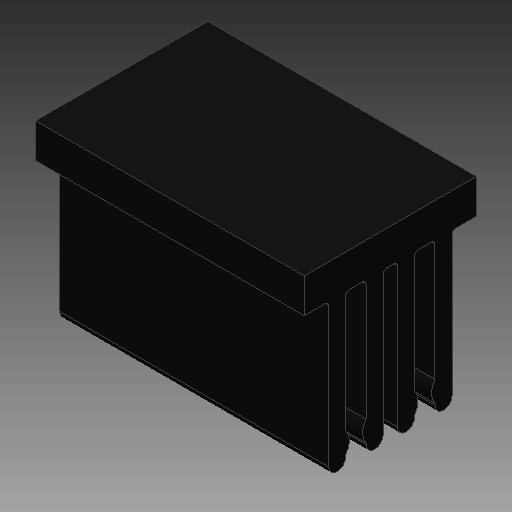
# Autodesk Inventor part: PPP-06-01-20--DV
Saved by Autodesk Inventor 2019.1 (Build 231200000, 200)
## iProperties
Category: PARTsolutions
Company: SAMTEC
Created: 2015-08-01
Part Number: PPP-06-01-20--DV
Catalog Web Link: www.cadenas.de
Description: TSM Series Pick & Place Pad-TSM Series - (2,54 mm) .100" Surface Mount Terminal .025" Square Post Header
Vendor: SAMTEC
Document SubType Name: Modeling
Designer: PARTuser1
Manufacturer: SAMTEC
Mass: 0.221539 g
Surface Area: 6.25221 cm^2
Volume: 0.221539 cm^3
Density: 1 g/cm^3
Material: Allgemein
Appearance: PSOLRGB-0-0-0
PSOL_IDENT_0: {$CADENAS_DATA\23d-libs\samtec\modelling\tsm\parts\tsm_ppp.prj},205 {VTYP=3D},{NB=PPP-06-01-20--DV},
PSOL_IDENT_1: {LINA=PPP-06-01-20--DV},{NN=TSM Series Pick & Place Pad},{DATE=15.05.2015 12:28:13},{GEOMDATE=25.09.
PSOL_IDENT_2: 2014 07:23:00},{VERSION=},{LINEID=10},{LINESUBID=-1},{WBVAR=LS,POS,ROW}  {NB=PPP-06-01-20--DV},{LINA=
PSOL_IDENT_3: PPP-06-01-20--DV},{KT=DUMMY},{PN=PPP-06-01-20--DV},{LS=-01},{POS=20},{ROW=-DV},{BSH=0.230},{CSH=0.18
PSOL_IDENT_4: 0},{ESH=0.1000},{ASH=0.9000},{POSOE=2},{BSV=0.230},{CSV=0.2800}
NN: TSM Series Pick & Place Pad
NT: TSM Series - (2,54 mm) .100" Surface Mount Terminal .025" Square Post Header
NB: PPP-06-01-20--DV
NBSYN: $PN.
LINA: PPP-06-01-20--DV
LS: -01
POS: 20
ROW: -DV - Double Vertical
SUPPLIER: SAMTEC
ARTICLENO: PPP-06-01-20--DV
BOMINFO: PPP-06-01-20--DV
CREATOR: CADENAS GmbH
Title: PPP-06-01-20--DV
Author: Cadenas PARTsolutions
Comments: TSM Series - (2,54 mm) .100" Surface Mount Terminal .025" Square Post Header
Autodesk Inventor part; units mm, degrees
sketch "Sketch_6" plane through (0, 0, 0) normal (1, 0, 0) x (0, 1, 0)
  line L0 (0, 3.175) -> (-1.27, 3.175)
  line L1 (-1.27, 3.175) -> (-1.27, 2.407)
  arc A0 (-1.397, 2.28) -> (-1.27, 2.407) centre (-1.397, 2.407) ccw
  line L2 (-1.397, 2.28) -> (-6.54, 2.28)
  arc A1 (-6.54, 2.28) -> (-6.54, 1.645) centre (-6.54, 1.9625) ccw
  line L3 (-6.54, 1.645) -> (-6.477, 1.645)
  arc A2 (-6.477, 1.645) -> (-5.715, 1.645) centre (-6.096, 2.153) ccw
  line L4 (-5.715, 1.645) -> (-1.397, 1.645)
  arc A3 (-1.27, 1.518) -> (-1.397, 1.645) centre (-1.397, 1.518) ccw
  line L5 (-1.27, 1.518) -> (-1.27, 1.022)
  arc A4 (-1.397, 0.895) -> (-1.27, 1.022) centre (-1.397, 1.022) ccw
  line L6 (-1.397, 0.895) -> (-5.715, 0.895)
  arc A5 (-5.715, 0.895) -> (-6.477, 0.895) centre (-6.096, 0.387) ccw
  line L7 (-6.477, 0.895) -> (-6.5222, 0.895)
  arc A6 (-6.5222, 0.895) -> (-6.5222, 0.26) centre (-6.5227, 0.5775) ccw
  line L8 (-6.5222, 0.26) -> (-1.397, 0.26)
  arc A7 (-1.27, 0.133) -> (-1.397, 0.26) centre (-1.397, 0.133) ccw
  line L9 (-1.27, 0.133) -> (-1.27, -0.133)
  arc A8 (-1.397, -0.26) -> (-1.27, -0.133) centre (-1.397, -0.133) ccw
  line L10 (-1.397, -0.26) -> (-6.54, -0.26)
  arc A9 (-6.54, -0.26) -> (-6.54, -0.895) centre (-6.54, -0.5775) ccw
  line L11 (-6.54, -0.895) -> (-6.477, -0.895)
  arc A10 (-6.477, -0.895) -> (-5.715, -0.895) centre (-6.096, -0.387) ccw
  line L12 (-5.715, -0.895) -> (-1.397, -0.895)
  arc A11 (-1.27, -1.022) -> (-1.397, -0.895) centre (-1.397, -1.022) ccw
  line L13 (-1.27, -1.022) -> (-1.27, -1.518)
  arc A12 (-1.397, -1.645) -> (-1.27, -1.518) centre (-1.397, -1.518) ccw
  line L14 (-1.397, -1.645) -> (-5.715, -1.645)
  arc A13 (-5.715, -1.645) -> (-6.477, -1.645) centre (-6.096, -2.153) ccw
  line L15 (-6.477, -1.645) -> (-6.54, -1.645)
  arc A14 (-6.54, -1.645) -> (-6.54, -2.28) centre (-6.54, -1.9625) ccw
  line L16 (-6.54, -2.28) -> (-1.397, -2.28)
  arc A15 (-1.27, -2.407) -> (-1.397, -2.28) centre (-1.397, -2.407) ccw
  line L17 (-1.27, -2.407) -> (-1.27, -3.175)
  line L18 (-1.27, -3.175) -> (0, -3.175)
  line L19 (0, -3.175) -> (0, 3.175)
  constraints: 40 end point, 32 point on circle, 16 centre point
extrude "Extrusion1" add sketch "Sketch_6" along normal mid plane 9.906
ref_plane "pick_place_pad_XY" through (0, 0, 0) normal (0, 1, 0) x (1, 0, 0)
ref_plane "pick_place_pad_YZ" through (0, 0, 0) normal (1, 0, 0) x (0, 0, -1)
ref_plane "pick_place_pad_ZX" through (0, 0, 0) normal (0, 0, -1) x (0, 1, 0)
body "Solid1"
